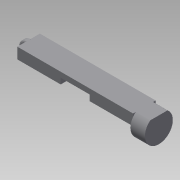
# Autodesk Inventor part: pig_nose_tail
Saved by Autodesk Inventor 2015 (Build 190159000, 159)
## iProperties
Created: 2016-04-29
Part Number: pig_nose_tail
Material: Generic
Document SubType Name: Modeling
Designer: Luke Good
Density: 1 g/cm^3
Appearance: Default
Author: Luke Good
Autodesk Inventor part; units mm, degrees
ref_plane "YZ Plane" through (0, 0, 0) normal (1, 0, 0) x (0, 1, 0)
ref_plane "XZ Plane" through (0, 0, 0) normal (0, 1, 0) x (-1, 0, 0)
ref_plane "XY Plane" through (0, 0, 0) normal (0, 0, 1) x (1, 0, 0)
sketch "Sketch1" plane through (0, 0, 0) normal (0, 1, 0) x (-1, 0, 0)
  line L0 (-25.4, 4.953) -> (25.4, 4.953)
  line L1 (25.4, 4.953) -> (25.4, -4.953)
  line L2 (25.4, -4.953) -> (-25.4, -4.953)
  line L3 (-25.4, -4.953) -> (-25.4, 4.953)
  line L4 (-25.4, 4.953) -> (25.4, -4.953) construction
  line L5 (25.4, 4.953) -> (-25.4, -4.953) construction
  point P0 (0, 0)
  dimension "d0" = 50.8
  dimension "d1" = 9.906
  constraints: 12 end point, 2 midpoint, 2 parallel, 1 horizontal, 1 perpendicular
  measures "d0" distance of L1.end L2.end
  measures "d1" distance of L0.end L1.end
extrude "Extrusion1" add sketch "Sketch1" along normal blind 4.826
sketch "Sketch2" plane through (-25.4, 0, 4.953) normal (0, 0, 1) x (1, 0, 0)
  line L0 (19.05, 0) -> (19.05, 2.54)
  line L1 (19.05, 2.54) -> (31.75, 2.54)
  line L2 (31.75, 2.54) -> (31.75, 0)
  line L3 (25.4, 0) -> (19.05, 2.54) construction
  line L4 (25.4, 0) -> (31.75, 2.54) construction
  line L5 (19.05, 0) -> (31.75, 0)
  line L6 (50.8, 0) -> (0, 0) projected
  point P0 (25.4, 0)
  constraints: 12 end point, 3 point on line, 1 midpoint, 1 parallel
extrude "Extrusion2" cut sketch "Sketch2" against normal blind 12.7
sketch "Sketch3" plane through (25.4, 0, 4.953) normal (1, 0, 0) x (0, 0, -1)
  arc A0 (1.1698, 4.826) -> (8.7362, 4.826) centre (4.953, 0) ccw
  line L0 (0, 4.826) -> (9.906, 4.826) projected
  line L1 (1.1698, 4.826) -> (8.7362, 4.826)
  constraints: 2 end point, 2 point on circle, 2 point on line, 1 centre point, 1 coincident
extrude "Extrusion3" add sketch "Sketch3" along normal blind 6.35
sketch "Sketch4" plane through (-25.4, 0, -4.953) normal (-1, 0, 0) x (0, 0, 1)
  point P0 (4.953, 0)
sketch "Sketch5" plane through (-25.4, 0, -4.953) normal (-1, 0, 0) x (0, 0, 1)
  arc A0 (4.1541, 4.8522) -> (5.7772, 4.826) centre (4.953, 4.0539) ccw
  line L0 (9.906, 1.595) -> (0, 1.595)
  line L1 (9.906, 0) -> (0, 0) projected
  line L2 (4.1541, 4.8522) -> (5.7772, 4.826)
  line L3 (1.1698, 4.826) -> (8.7362, 4.826) projected
  point P0 (4.953, 0)
  constraints: 4 end point, 2 point on circle, 1 centre point, 1 parallel, 1 point on line
revolve "Revolution1" add sketch "Sketch5" angle 90 about axis through (-25.4, 1.595, 4.953) along (0, 0, 1)
body "Solid1"
